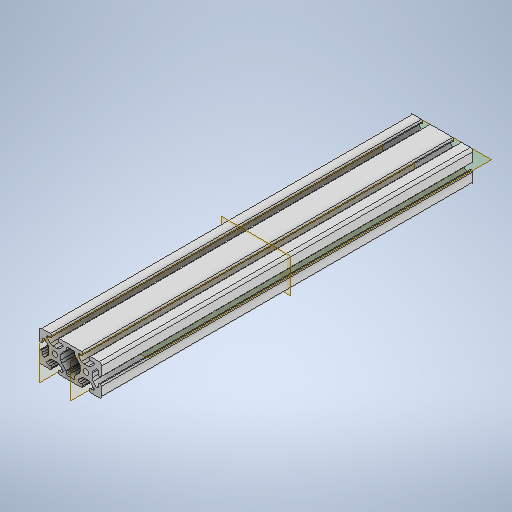
# Autodesk Inventor part: 4080_Y_BASE
Saved by Autodesk Inventor 2025.2 (Build 292293000, 293)
## iProperties
Created: 2026-02-05
Part Number: 4080_Y_BASE
Material: Generic
Document SubType Name: Modeling
Designer: composite
Density: 1 g/cm^3
Appearance: Default
Author: composite
Autodesk Inventor part; units mm, degrees
ref_plane "YZ Plane" through (0, 0, 0) normal (1, 0, 0) x (0, 1, 0)
ref_plane "XZ Plane" through (0, 0, 0) normal (0, 1, 0) x (-1, 0, 0)
ref_plane "XY Plane" through (0, 0, 0) normal (0, 0, 1) x (1, 0, 0)
derived "4080_REPRESENTATIVE.ipt"
sketch "Sketch1" plane through (-14.3719, 20, 0) normal (0, 0, 1) x (1, 0, 0)
  arc A0 (28.7419, -40) -> (30.3119, -38.43) centre (28.7419, -38.43) ccw
  line L0 (30.3119, -38.43) -> (30.3119, -37.25)
  arc A1 (30.3119, -37.25) -> (28.7419, -35.68) centre (28.7419, -37.25) ccw
  line L1 (28.7419, -35.68) -> (25.6569, -35.68)
  arc A2 (24.0869, -34.11) -> (25.6569, -35.68) centre (25.6569, -34.11) ccw
  line L2 (24.0869, -34.11) -> (24.0869, -33.6545)
  arc A3 (24.3095, -33.1171) -> (24.0869, -33.6545) centre (24.8469, -33.6545) ccw
  line L3 (24.3095, -33.1171) -> (28.0624, -29.3642)
  arc A4 (31.0303, -27.7) -> (28.0624, -29.3642) centre (31.7154, -32.4003) ccw
  line L4 (31.0303, -27.7) -> (37.7134, -27.7)
  arc A5 (40.6814, -29.3642) -> (37.7134, -27.7) centre (37.0284, -32.4003) ccw
  line L5 (40.6814, -29.3642) -> (44.4343, -33.1171)
  arc A6 (44.6569, -33.6545) -> (44.4343, -33.1171) centre (43.8969, -33.6545) ccw
  line L6 (44.6569, -33.6545) -> (44.6569, -34.11)
  arc A7 (43.0869, -35.68) -> (44.6569, -34.11) centre (43.0869, -34.11) ccw
  line L7 (43.0869, -35.68) -> (40.0019, -35.68)
  arc A8 (40.0019, -35.68) -> (38.4319, -37.25) centre (40.0019, -37.25) ccw
  line L8 (38.4319, -37.25) -> (38.4319, -38.4389)
  arc A9 (38.4319, -38.4389) -> (40.1689, -40) centre (40.0019, -38.4389) ccw
  line L9 (40.1689, -40) -> (51.4293, -40)
  arc A10 (51.4293, -40) -> (54.3719, -36.83) centre (51.2019, -36.8382) ccw
  line L10 (54.3719, -36.83) -> (54.3719, -25.5696)
  arc A11 (54.3719, -25.5696) -> (52.8019, -24.06) centre (52.8031, -25.63) ccw
  line L11 (52.8019, -24.06) -> (51.6219, -24.06)
  arc A12 (51.6219, -24.06) -> (50.0519, -25.63) centre (51.6219, -25.63) ccw
  line L12 (50.0519, -25.63) -> (50.0519, -28.715)
  arc A13 (48.4829, -30.3398) -> (50.0519, -28.715) centre (48.4829, -28.7698) ccw
  line L13 (48.4829, -30.3398) -> (48.0812, -30.3398)
  arc A14 (47.5438, -30.1172) -> (48.0812, -30.3398) centre (48.0812, -29.5798) ccw
  line L14 (47.5438, -30.1172) -> (43.2874, -25.8608)
  arc A15 (42.0878, -22.502) -> (43.2874, -25.8608) centre (46.8336, -22.7006) ccw
  line L15 (42.0878, -22.502) -> (42.0878, -17.429)
  arc A16 (43.383, -14.0436) -> (42.0878, -17.429) centre (46.8361, -17.3052) ccw
  line L16 (43.383, -14.0436) -> (47.4854, -9.9412)
  arc A17 (48.0228, -9.7186) -> (47.4854, -9.9412) centre (48.0228, -10.4786) ccw
  line L17 (48.0228, -9.7186) -> (48.4819, -9.7186)
  arc A18 (50.0519, -11.2886) -> (48.4819, -9.7186) centre (48.4819, -11.2886) ccw
  line L18 (50.0519, -11.2886) -> (50.0519, -14.3736)
  arc A19 (50.0519, -14.3736) -> (51.5162, -15.94) centre (51.6219, -14.3736) ccw
  line L19 (51.5162, -15.94) -> (52.6962, -15.94)
  arc A20 (52.6962, -15.94) -> (54.3719, -14.4175) centre (52.8025, -14.3736) ccw
  line L20 (54.3719, -14.4175) -> (54.3719, -3.1594)
  arc A21 (54.3719, -3.1594) -> (51.2019, 0) centre (51.2019, -3.17) ccw
  line L21 (51.2019, 0) -> (39.9414, 0)
  arc A22 (39.9414, 0) -> (38.4319, -1.5688) centre (40.0019, -1.5688) ccw
  line L22 (38.4319, -1.5688) -> (38.4319, -2.75)
  arc A23 (38.4319, -2.75) -> (40.0019, -4.32) centre (40.0019, -2.75) ccw
  line L23 (40.0019, -4.32) -> (43.0869, -4.32)
  arc A24 (44.6569, -5.89) -> (43.0869, -4.32) centre (43.0869, -5.89) ccw
  line L24 (44.6569, -5.89) -> (44.6569, -6.3455)
  arc A25 (44.4343, -6.8829) -> (44.6569, -6.3455) centre (43.8969, -6.3455) ccw
  line L25 (44.4343, -6.8829) -> (40.28, -11.0372)
  arc A26 (36.9213, -12.3) -> (40.28, -11.0372) centre (37.0528, -7.5518) ccw
  line L26 (36.9213, -12.3) -> (31.8225, -12.3)
  arc A27 (28.4638, -11.0372) -> (31.8225, -12.3) centre (31.691, -7.5518) ccw
  line L27 (28.4638, -11.0372) -> (24.3095, -6.8829)
  arc A28 (24.0869, -6.3455) -> (24.3095, -6.8829) centre (24.8469, -6.3455) ccw
  line L28 (24.0869, -6.3455) -> (24.0869, -5.89)
  arc A29 (25.6569, -4.32) -> (24.0869, -5.89) centre (25.6569, -5.89) ccw
  line L29 (25.6569, -4.32) -> (28.7419, -4.32)
  arc A30 (28.7419, -4.32) -> (30.3119, -2.8271) centre (28.7438, -2.75) ccw
  line L30 (30.3119, -2.8271) -> (30.3119, -1.6471)
  arc A31 (30.3119, -1.6471) -> (28.7438, 0) centre (28.7438, -1.57) ccw
  line L31 (28.7438, 0) -> (0, 0)
  arc A32 (0, 0) -> (-1.5681, -1.6471) centre (0, -1.57) ccw
  line L32 (-1.5681, -1.6471) -> (-1.5681, -2.8271)
  arc A33 (-1.5681, -2.8271) -> (0.0019, -4.32) centre (0, -2.75) ccw
  line L33 (0.0019, -4.32) -> (3.0869, -4.32)
  arc A34 (4.6569, -5.89) -> (3.0869, -4.32) centre (3.0869, -5.89) ccw
  line L34 (4.6569, -5.89) -> (4.6569, -6.3455)
  arc A35 (4.4343, -6.8829) -> (4.6569, -6.3455) centre (3.8969, -6.3455) ccw
  line L35 (4.4343, -6.8829) -> (0.28, -11.0372)
  arc A36 (-3.0787, -12.3) -> (0.28, -11.0372) centre (-2.9472, -7.5518) ccw
  line L36 (-3.0787, -12.3) -> (-8.1775, -12.3)
  arc A37 (-11.5362, -11.0372) -> (-8.1775, -12.3) centre (-8.309, -7.5518) ccw
  line L37 (-11.5362, -11.0372) -> (-15.6905, -6.8829)
  arc A38 (-15.9131, -6.3455) -> (-15.6905, -6.8829) centre (-15.1531, -6.3455) ccw
  line L38 (-15.9131, -6.3455) -> (-15.9131, -5.89)
  arc A39 (-14.3431, -4.32) -> (-15.9131, -5.89) centre (-14.3431, -5.89) ccw
  line L39 (-14.3431, -4.32) -> (-11.2581, -4.32)
  arc A40 (-11.2581, -4.32) -> (-9.6881, -2.75) centre (-11.2581, -2.75) ccw
  line L40 (-9.6881, -2.75) -> (-9.6881, -1.5688)
  arc A41 (-9.6881, -1.5688) -> (-11.1977, 0) centre (-11.2581, -1.5688) ccw
  line L41 (-11.1977, 0) -> (-22.4581, 0)
  arc A42 (-22.4581, 0) -> (-25.6281, -3.1594) centre (-22.4581, -3.17) ccw
  line L42 (-25.6281, -3.1594) -> (-25.6281, -14.4175)
  arc A43 (-25.6281, -14.4175) -> (-23.9524, -15.94) centre (-24.0587, -14.3736) ccw
  line L43 (-23.9524, -15.94) -> (-22.7724, -15.94)
  arc A44 (-22.7724, -15.94) -> (-21.3081, -14.3736) centre (-22.8781, -14.3736) ccw
  line L44 (-21.3081, -14.3736) -> (-21.3081, -11.2886)
  arc A45 (-19.7381, -9.7186) -> (-21.3081, -11.2886) centre (-19.7381, -11.2886) ccw
  line L45 (-19.7381, -9.7186) -> (-19.279, -9.7186)
  arc A46 (-18.7416, -9.9412) -> (-19.279, -9.7186) centre (-19.279, -10.4786) ccw
  line L46 (-18.7416, -9.9412) -> (-14.6392, -14.0436)
  arc A47 (-13.344, -17.429) -> (-14.6392, -14.0436) centre (-18.0924, -17.3052) ccw
  line L47 (-13.344, -17.429) -> (-13.344, -22.502)
  arc A48 (-14.5436, -25.8608) -> (-13.344, -22.502) centre (-18.0898, -22.7006) ccw
  line L48 (-14.5436, -25.8608) -> (-18.8, -30.1172)
  arc A49 (-19.3374, -30.3398) -> (-18.8, -30.1172) centre (-19.3374, -29.5798) ccw
  line L49 (-19.3374, -30.3398) -> (-19.7391, -30.3398)
  arc A50 (-21.3081, -28.715) -> (-19.7391, -30.3398) centre (-19.7391, -28.7698) ccw
  line L50 (-21.3081, -28.715) -> (-21.3081, -25.63)
  arc A51 (-21.3081, -25.63) -> (-22.8781, -24.06) centre (-22.8781, -25.63) ccw
  line L51 (-22.8781, -24.06) -> (-24.0581, -24.06)
  arc A52 (-24.0581, -24.06) -> (-25.6281, -25.5696) centre (-24.0593, -25.63) ccw
  line L52 (-25.6281, -25.5696) -> (-25.6281, -36.83)
  arc A53 (-25.6281, -36.83) -> (-22.6855, -40) centre (-22.4581, -36.8382) ccw
  line L53 (-22.6855, -40) -> (-11.4251, -40)
  arc A54 (-11.4251, -40) -> (-9.6881, -38.4389) centre (-11.2581, -38.4389) ccw
  line L54 (-9.6881, -38.4389) -> (-9.6881, -37.25)
  arc A55 (-9.6881, -37.25) -> (-11.2581, -35.68) centre (-11.2581, -37.25) ccw
  line L55 (-11.2581, -35.68) -> (-14.3431, -35.68)
  arc A56 (-15.9131, -34.11) -> (-14.3431, -35.68) centre (-14.3431, -34.11) ccw
  line L56 (-15.9131, -34.11) -> (-15.9131, -33.6545)
  arc A57 (-15.6905, -33.1171) -> (-15.9131, -33.6545) centre (-15.1531, -33.6545) ccw
  line L57 (-15.6905, -33.1171) -> (-11.9376, -29.3642)
  arc A58 (-8.9697, -27.7) -> (-11.9376, -29.3642) centre (-8.2846, -32.4003) ccw
  line L58 (-8.9697, -27.7) -> (-2.2866, -27.7)
  arc A59 (0.6814, -29.3642) -> (-2.2866, -27.7) centre (-2.9716, -32.4003) ccw
  line L59 (0.6814, -29.3642) -> (4.4343, -33.1171)
  arc A60 (4.6569, -33.6545) -> (4.4343, -33.1171) centre (3.8969, -33.6545) ccw
  line L60 (4.6569, -33.6545) -> (4.6569, -34.11)
  arc A61 (3.0869, -35.68) -> (4.6569, -34.11) centre (3.0869, -34.11) ccw
  line L61 (3.0869, -35.68) -> (0.0019, -35.68)
  arc A62 (0.0019, -35.68) -> (-1.5681, -37.25) centre (0.0019, -37.25) ccw
  line L62 (-1.5681, -37.25) -> (-1.5681, -38.43)
  arc A63 (-1.5681, -38.43) -> (0.0019, -40) centre (0.0019, -38.43) ccw
  line L63 (0.0019, -40) -> (28.7419, -40)
  circle A64 centre (34.3719, -20) radius 3.4
  line L64 (3.1707, -25.7441) -> (8.6582, -31.2316)
  arc A65 (2.0878, -22.725) -> (3.1707, -25.7441) centre (6.8378, -22.725) ccw
  line L65 (2.0878, -16.7409) -> (2.0878, -22.725)
  arc A66 (3.7731, -13.6535) -> (2.0878, -16.7409) centre (6.8034, -17.3113) ccw
  line L66 (8.6582, -8.7684) -> (3.7731, -13.6535)
  arc A67 (8.6582, -8.7684) -> (9.0301, -7.8704) centre (7.7601, -7.8704) ccw
  line L67 (9.0301, -5.59) -> (9.0301, -7.8704)
  arc A68 (10.3001, -4.32) -> (9.0301, -5.59) centre (10.3001, -5.59) ccw
  line L68 (18.4436, -4.32) -> (10.3001, -4.32)
  arc A69 (19.7136, -5.59) -> (18.4436, -4.32) centre (18.4436, -5.59) ccw
  line L69 (19.7136, -7.8704) -> (19.7136, -5.59)
  arc A70 (19.7136, -7.8704) -> (20.0856, -8.7684) centre (20.9836, -7.8704) ccw
  line L70 (24.9707, -13.6535) -> (20.0856, -8.7684)
  arc A71 (26.656, -16.7409) -> (24.9707, -13.6535) centre (21.9404, -17.3113) ccw
  line L71 (26.656, -22.725) -> (26.656, -16.7409)
  arc A72 (25.5731, -25.7441) -> (26.656, -22.725) centre (21.906, -22.725) ccw
  line L72 (20.0856, -31.2316) -> (25.5731, -25.7441)
  arc A73 (20.0856, -31.2316) -> (19.7136, -32.1296) centre (20.9836, -32.1296) ccw
  line L73 (19.7136, -34.41) -> (19.7136, -32.1296)
  arc A74 (18.4436, -35.68) -> (19.7136, -34.41) centre (18.4436, -34.41) ccw
  line L74 (10.3001, -35.68) -> (18.4436, -35.68)
  arc A75 (9.0301, -34.41) -> (10.3001, -35.68) centre (10.3001, -34.41) ccw
  line L75 (9.0301, -32.1296) -> (9.0301, -34.41)
  arc A76 (9.0301, -32.1296) -> (8.6582, -31.2316) centre (7.7601, -32.1296) ccw
  circle A77 centre (-5.6281, -20) radius 3.4
  point P0 (14.3719, -20)
extrude "Extrusion1" add sketch "Sketch1" along normal blind 475
ref_plane "Work Plane1" through (-14.37, 0, 0) normal (0, -1, 0) x (1, 0, 0)
ref_plane "Work Plane2" through (-14.3719, 20, 237.5) normal (0, 0, 1) x (1, 0, 0)
ref_plane "Work Plane3" through (20, -17.25, 475) normal (1, 0, 0) x (0, 0, -1)
ref_plane "Work Plane4" through (-20, -17.25, 475) normal (1, 0, 0) x (0, 0, -1)
body "Solid1"
